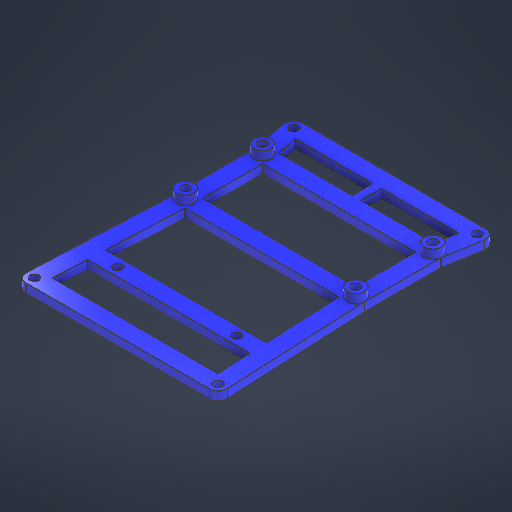
# Autodesk Inventor part: bigbucksupport
Saved by Autodesk Inventor 2026.1 (Build 301233000, 233)
## iProperties
Created: 2026-04-25
Part Number: bigbucksupport
Material: Generic
Document SubType Name: Modeling
Designer: emanuel
Density: 1 g/cm^3
Appearance: Default
Author: emanuel
Autodesk Inventor part; units mm, degrees
ref_plane "YZ Plane" through (0, 0, 0) normal (1, 0, 0) x (0, 1, 0)
ref_plane "XZ Plane" through (0, 0, 0) normal (0, 1, 0) x (-1, 0, 0)
ref_plane "XY Plane" through (0, 0, 0) normal (0, 0, 1) x (1, 0, 0)
sketch "Sketch1" plane through (0, 0, 0) normal (0, 1, 0) x (-1, 0, 0)
  line L0 (0, 0) -> (58.5, 0)
  line L1 (58.5, 0) -> (58.5, -26.5)
  line L2 (58.5, -26.5) -> (0, -26.5)
  line L3 (0, -26.5) -> (0, 0)
  circle A0 centre (58.5, 0) radius 1.5
  circle A1 centre (58.5, -26.5) radius 1.5
  circle A2 centre (0, 0) radius 1.5
  circle A3 centre (0, -26.5) radius 1.5
  circle A4 centre (0, 0) radius 3
  circle A5 centre (0, -26.5) radius 3
  circle A6 centre (58.5, 0) radius 3
  circle A7 centre (58.5, -26.5) radius 3
  dimension "d0" = 58.5
  dimension "d1" = 26.5
  dimension "d2" = 3
  dimension "d3" = 3
  dimension "d4" = 3
  dimension "d5" = 3
  dimension "d6" = 6
  dimension "d7" = 6
  dimension "d8" = 6
  dimension "d9" = 6
  constraints: 8 centre point, 8 coincident, 8 end point, 2 parallel, 1 horizontal, 1 perpendicular
  measures "d0" distance of L1.end L2.end
  measures "d1" distance of L0.end L1.end
  measures "d2" diameter of A0
  measures "d3" diameter of A1
  measures "d4" diameter of A2
  measures "d5" diameter of A3
  measures "d6" diameter of A4
  measures "d7" diameter of A5
  measures "d8" diameter of A6
  measures "d9" diameter of A7
extrude "Extrusion1" add sketch "Sketch1" along normal blind 3 contours A2 L3 A4 L0 | L0 A4 L3 A2 | A6 L1 A0 L0 | L0 A0 L1 A6 | A5 L2 A3 L3 | L3 A3 L2 A5 | A7 L2 A1 L1 | L1 A1 L2 A7
sketch "Sketch2" plane through (0, 0, 0) normal (0, -1, 0) x (1, 0, 0)
  circle A0 centre (0, 0) radius 1.5
  circle A1 centre (0, -26.5) radius 1.5 projected
  circle A2 centre (0, -26.5) radius 1.5
  circle A3 centre (-58.5, -26.5) radius 1.5 projected
  circle A4 centre (-58.5, -26.5) radius 1.5
  circle A5 centre (-58.5, 0) radius 1.5 projected
  circle A6 centre (-58.5, 0) radius 1.5
  line L0 (-58.5, 0) -> (0, 0) construction
  line L1 (-58.5, -3) -> (0, -3)
  line L2 (0, 3) -> (-58.5, 3)
  arc A7 (-58.5, 3) -> (-58.5, -3) centre (-58.5, 0) ccw
  arc A8 (0, -3) -> (0, 3) centre (0, 0) ccw
  line L3 (0, 0) -> (0, -26.5) construction
  line L4 (-3, 0) -> (-3, -26.5)
  line L5 (3, -26.5) -> (3, 0)
  arc A9 (3, 0) -> (-3, 0) centre (0, 0) ccw
  arc A10 (-3, -26.5) -> (3, -26.5) centre (0, -26.5) ccw
  line L6 (0, -26.5) -> (-58.5, -26.5) construction
  line L7 (0, -29.5) -> (-58.5, -29.5)
  line L8 (-58.5, -23.5) -> (0, -23.5)
  arc A11 (0, -29.5) -> (0, -23.5) centre (0, -26.5) ccw
  arc A12 (-58.5, -23.5) -> (-58.5, -29.5) centre (-58.5, -26.5) ccw
  line L9 (-58.5, -26.5) -> (-58.5, 0) construction
  line L10 (-55.5, -26.5) -> (-55.5, 0)
  line L11 (-61.5, 0) -> (-61.5, -26.5)
  arc A13 (-61.5, -26.5) -> (-55.5, -26.5) centre (-58.5, -26.5) ccw
  arc A14 (-55.5, 0) -> (-61.5, 0) centre (-58.5, 0) ccw
  point P0 (-29.25, 0)
  point P1 (0, -13.25)
  point P2 (-29.25, -26.5)
  point P3 (-58.5, -13.25)
  point P4 (-3, -3)
  point P5 (-3, -23.5)
  point P6 (-55.5, -23.5)
  point P7 (-55.5, -3)
  constraints: 32 end point, 16 point on circle, 16 tangent, 12 centre point, 4 coincident, 4 midpoint, 4 parallel, 3 perpendicular, 1 horizontal
extrude "Extrusion2" add sketch "Sketch2" along normal blind 3 contours A7 A14 L10 L1 | L1 L10 L8 A12 L11 A7 | L10 A14 L2 A9 L4 L1 | L4 A9 A8 L1 | L1 A8 L5 A11 L8 L4 | L10 A13 A12 L8 | L8 L4 A10 L7 A13 L10 | L8 A11 A10 L4
sketch "Sketch3" plane through (0, -3, 0) normal (0, -1, 0) x (1, 0, 0)
  line L0 (-58.5, -29.5) -> (0, -29.5) projected
  line L1 (-29.25, -29.5) -> (-29.25, -39.5)
  line L2 (-60.75, -39.5) -> (2.25, -39.5)
  circle A0 centre (-60.75, -39.5) radius 1.5
  circle A1 centre (2.25, -39.5) radius 1.5
  circle A2 centre (-58.5, -26.5) radius 1.5 projected
  line L3 (-60.75, -39.5) -> (-58.5, -26.5) construction
  line L4 (-57.7939, -40.0116) -> (-55.5439, -27.0116)
  line L5 (-61.4561, -25.9884) -> (-63.7061, -38.9884)
  arc A3 (-63.7061, -38.9884) -> (-57.7939, -40.0116) centre (-60.75, -39.5) ccw
  arc A4 (-55.5439, -27.0116) -> (-61.4561, -25.9884) centre (-58.5, -26.5) ccw
  circle A5 centre (0, -26.5) radius 1.5 projected
  line L6 (2.25, -39.5) -> (0, -26.5) construction
  line L7 (5.2061, -38.9884) -> (2.9561, -25.9884)
  line L8 (-2.9561, -27.0116) -> (-0.7061, -40.0116)
  arc A6 (-0.7061, -40.0116) -> (5.2061, -38.9884) centre (2.25, -39.5) ccw
  arc A7 (2.9561, -25.9884) -> (-2.9561, -27.0116) centre (0, -26.5) ccw
  line L9 (-60.75, -39.5) -> (2.25, -39.5) construction
  line L10 (-60.75, -36.5) -> (2.25, -36.5)
  line L11 (2.25, -42.5) -> (-60.75, -42.5)
  arc A8 (-60.75, -36.5) -> (-60.75, -42.5) centre (-60.75, -39.5) ccw
  arc A9 (2.25, -42.5) -> (2.25, -36.5) centre (2.25, -39.5) ccw
  line L12 (-29.25, -39.5) -> (-29.25, -27.0116) construction
  line L13 (-27.75, -39.5) -> (-27.75, -27.0116)
  line L14 (-30.75, -27.0116) -> (-30.75, -39.5)
  arc A10 (-30.75, -39.5) -> (-27.75, -39.5) centre (-29.25, -39.5) ccw
  arc A11 (-27.75, -27.0116) -> (-30.75, -27.0116) centre (-29.25, -27.0116) ccw
  point P0 (0, 0)
  point P1 (-59.625, -33)
  point P2 (1.125, -33)
  point P3 (-29.25, -33.2558)
  point P4 (-57.1862, -36.5)
  point P5 (-1.3138, -36.5)
  point P6 (-27.75, -36.5)
  point P7 (-30.75, -36.5)
  dimension "d14" = 10
  dimension "d15" = 63
  dimension "d16" = 3
  dimension "d17" = 3
  dimension "d18" = 6
  dimension "d19" = 6
  dimension "d20" = 3
  constraints: 36 end point, 16 point on circle, 16 tangent, 10 centre point, 6 midpoint, 5 equal length, 2 coincident, 1 concentric, 1 horizontal, 1 point on line, 1 vertical
  measures "d14" distance of L1.start L1.end
  measures "d15" distance of L2.start L2.end
  measures "d16" diameter of A0
  measures "d17" diameter of A1
  measures "d18" diameter of A4
  measures "d19" diameter of A7
  measures "d20" diameter of A11
extrude "Extrusion3" add sketch "Sketch3" against normal blind 3 contours L4 L10 A8 L5 A4 | L14 A11 L13 L0 | L0 L1 L10 L14 | L10 L14 L2 L4 | L4 A3 A8 L10 | L0 L13 L10 L1 | L10 L1 L2 L14 | L2 A10 L8 A6 L11 A3 L4 | L10 L13 L2 L1 | L2 A10 | L8 A7 L7 A9 L10 | L10 L8 L2 L13 | L10 A9 A6 L8
sketch "Sketch4" plane through (0, 0, 0) normal (0, 1, 0) x (1, 0, 0)
  circle A0 centre (2.25, 39.5) radius 1.5 projected
  line L0 (2.25, 39.5) -> (2.25, -49.5)
  line L1 (2.25, -49.5) -> (-60.75, -49.5)
  circle A1 centre (2.25, -49.5) radius 1.5
  circle A2 centre (-60.75, -49.5) radius 1.5
  circle A3 centre (-58.5, 0) radius 1.5 projected
  line L2 (-60.75, -49.5) -> (-58.5, 0) construction
  line L3 (-57.7531, -49.6362) -> (-55.5031, -0.1362)
  line L4 (-61.4969, 0.1362) -> (-63.7469, -49.3638)
  arc A4 (-63.7469, -49.3638) -> (-57.7531, -49.6362) centre (-60.75, -49.5) ccw
  arc A5 (-55.5031, -0.1362) -> (-61.4969, 0.1362) centre (-58.5, 0) ccw
  line L5 (2.25, -49.5) -> (0, 0) construction
  line L6 (5.2469, -49.3638) -> (2.9969, 0.1362)
  line L7 (-2.9969, -0.1362) -> (-0.7469, -49.6362)
  arc A6 (-0.7469, -49.6362) -> (5.2469, -49.3638) centre (2.25, -49.5) ccw
  arc A7 (2.9969, 0.1362) -> (-2.9969, -0.1362) centre (0, 0) ccw
  line L8 (2.25, -49.5) -> (-60.75, -49.5) construction
  line L9 (2.25, -46.5) -> (-60.75, -46.5)
  line L10 (-60.75, -52.5) -> (2.25, -52.5)
  arc A8 (2.25, -52.5) -> (2.25, -46.5) centre (2.25, -49.5) ccw
  arc A9 (-60.75, -46.5) -> (-60.75, -52.5) centre (-60.75, -49.5) ccw
  circle A10 centre (0, 0) radius 1.5
  circle A11 centre (-58.5, 0) radius 1.5
  point P0 (-59.625, -24.75)
  point P1 (1.125, -24.75)
  point P2 (-29.25, -49.5)
  point P3 (-0.8895, -46.5)
  point P4 (-57.6105, -46.5)
  point P5 (2.25, -52.5)
  dimension "d23" = 89
  dimension "d24" = 63
  dimension "d25" = 3
  dimension "d26" = 3
  dimension "d27" = 6
  dimension "d28" = 6
  constraints: 28 end point, 12 point on circle, 12 tangent, 10 centre point, 4 coincident, 3 midpoint, 3 parallel, 2 perpendicular, 1 vertical
  measures "d23" distance of L0.start L0.end
  measures "d24" distance of L0.end L1.end
  measures "d25" diameter of A1
  measures "d26" diameter of A2
  measures "d27" diameter of A5
  measures "d28" diameter of A7
extrude "Extrusion4" add sketch "Sketch4" against normal blind 3 contours A7 L6 A8 L0 | L0 L9 L7 A7 | A8 A6 L7 L1 A1 L0 | L0 A1 L1 L7 L9 | L7 L1 L3 L9 | L7 A6 L10 A4 L3 L1 | L9 A9 L4 A5 L3 | L3 A4 A9 L9
sketch "Sketch5" plane through (0, 0, 0) normal (0, 1, 0) x (1, 0, 0)
  circle A0 centre (-58.5, 0) radius 1.5 projected
  line L0 (-58.5, 0) -> (0, 0)
  line L1 (0, 0) -> (0, -35)
  line L2 (0, -35) -> (-58.5, -35)
  line L3 (-58.5, -35) -> (-58.5, 0)
  line L4 (0, -35) -> (-58.5, -35)
  line L5 (-58.5, -35) -> (-58.5, -29)
  line L6 (-58.5, -29) -> (0, -29)
  line L7 (0, -29) -> (0, -35)
  line L8 (-29.25, -29) -> (-29.25, -35)
  line L9 (-49.672, -32) -> (-8.828, -32)
  circle A1 centre (-49.672, -32) radius 1.5
  circle A2 centre (-8.828, -32) radius 1.5
  point P0 (-29.25, -32)
  point P1 (0, -29)
  dimension "d31" = 35
  dimension "d32" = 6
  dimension "d33" = 40.844
  dimension "d34" = 3
  dimension "d35" = 3
  constraints: 20 end point, 4 midpoint, 4 parallel, 3 horizontal, 2 centre point, 2 coincident, 2 perpendicular, 1 point on line
  measures "d31" distance of L0.end L1.end
  measures "d32" distance of L4.end L5.end
  measures "d33" distance of L9.start L9.end
  measures "d34" diameter of A1
  measures "d35" diameter of A2
extrude "Extrusion5" add sketch "Sketch5" against normal blind 3 contours L6 L8 L2 L3 | L1 L2 L8 L6
body "Solid1"
